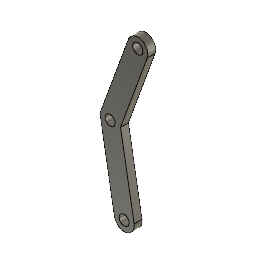
default (Autodesk Fusion 360 archive; units mm, degrees)
design "linkage2"
Autodesk Fusion 360 part; units mm, degrees
sketch "Sketch1" plane through (0, 0, 0) normal (0, 1, 0) x (1, 0, 0)
  line L0 (0, 0) -> (-735.0705, 0) construction
  line L1 (0, 0) -> (-636.5897, -367.5353) construction
  line L2 (0, 0) -> (-735.0705, -196.9616) construction
  circle A0 centre (-735.0705, -196.9616) radius 25
  circle A1 centre (-735.0705, -196.9616) radius 12.5
  circle A2 centre (-700.3409, 0) radius 25
  circle A3 centre (-700.3409, 0) radius 12.5
  circle A4 centre (-666.6665, -384.9001) radius 25
  circle A5 centre (-666.6665, -384.9001) radius 12.5
  line L3 (-675.7207, -4.3412) -> (-710.4503, -201.3028)
  line L4 (-759.6907, -192.6203) -> (-724.9611, 4.3412)
  line L5 (-643.1742, -376.3496) -> (-711.5782, -188.411)
  line L6 (-690.1588, -393.4506) -> (-758.5628, -205.5121)
  line L7 (-666.6665, -384.9001) -> (-735.0705, -196.9616) construction
  line L8 (-735.0705, -196.9616) -> (-700.3409, 0) construction
  line L9 (-735.0705, -196.9616) -> (-735.0705, 0) construction
  line L10 (-735.0705, -196.9616) -> (-636.5897, -367.5353) construction
  dimension "d2" = 30
  dimension "d3" = 15
  dimension "d6" = 50
  dimension "d7" = 25
  dimension "d8" = 50
  dimension "d9" = 25
  dimension "d10" = 50
  dimension "d11" = 25
  dimension "d15" = 10
  dimension "d16" = 10
  dimension "d17" = 200
  measures "d2" angle of L0 L1
  measures "d3" angle of L0 L2
  measures "d6" diameter of A0
  measures "d7" diameter of A1
  measures "d8" diameter of A4
  measures "d9" diameter of A5
  measures "d10" diameter of A2
  measures "d11" diameter of A3
  measures "d15" angle of L8 L9
  measures "d16" angle of L7 L10
extrude "Extrude1" add sketch "Sketch1" along normal mid plane 20
equation "d3 = d2 / 2"
equation "d7 = d6 / 2"
equation "d8 = d6"
equation "d9 = d7"
equation "d10 = d6"
equation "d11 = d7"
equation "d16 = d15"

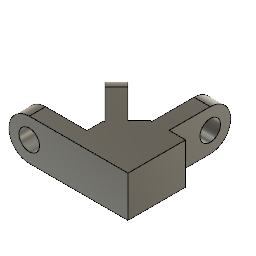
design "node2"
Autodesk Fusion 360 part; units mm, degrees
sketch "Sketch1" plane through (0, 0, 0) normal (0, 1, 0) x (1, 0, 0)
  circle A0 centre (-100, 0) radius 12.5
  circle A1 centre (100, 0) radius 12.5
  line L0 (100, 0) -> (-100, 0) construction
  circle A2 centre (-100, 0) radius 25
  circle A3 centre (100, 0) radius 25
  line L1 (100, -25) -> (-100, -25)
  line L2 (100, 25) -> (-100, 25)
  dimension "d1" = 200
  dimension "d2" = 25
  dimension "d3" = 25
  dimension "d4" = 12.5
  measures "d2" diameter of A0
  measures "d3" diameter of A1
  measures "d4" distance of A0 A2
extrude "Extrude1" add sketch "Sketch1" along normal mid plane 40 makes body 1
sketch "Sketch2" plane through (0, 0, 0) normal (1, 0, 0) x (0, 1, 0)
  circle A0 centre (100, 0) radius 12.5
  circle A1 centre (-100, 0) radius 12.5
  line L0 (100, 0) -> (-100, 0) construction
  circle A2 centre (-100, 0) radius 25
  circle A3 centre (100, 0) radius 25
  line L1 (100, 25) -> (-100, 25)
  line L2 (100, -25) -> (-100, -25)
  dimension "d8" = 200
  dimension "d9" = 25
  dimension "d10" = 25
  dimension "d11" = 12.5
  measures "d9" diameter of A1
  measures "d10" diameter of A0
  measures "d11" distance of A1 A2
extrude "Extrude2" add sketch "Sketch2" along normal mid plane 40 bodies 1
pattern_circular "C-Pattern1" count 2 over 45 about axis through (0, 0, 1.75) along (0, 0, 1) of bodies 1 makes body 2
sketch "Sketch3" plane through (0, 0, 0) normal (0, 0, 1) x (1, 0, 0)
  circle A0 centre (0, 0) radius 169.3734
  line L0 (20, -20) -> (-168.1884, -20)
  line L1 (20, -20) -> (20, 168.1884)
extrude "Extrude3" cut sketch "Sketch3" along normal mid plane 60 contours A0 L0 L1 picked at (28.044, 103.9038) bodies 1 2
combine "Combine1" operation add target body 1 tool bodies 2
sketch "Sketch4" plane through (0, 0, 0) normal (0, 1, 0) x (1, 0, 0)
  circle A0 centre (-100, 0) radius 25
  circle A1 centre (-100, 0) radius 12.5
  line L0 (-100, 25) -> (-50, 25)
  line L1 (-50, 25) -> (-50, -25)
  line L2 (-50, -25) -> (-100, -25)
  dimension "d18" = 50
  dimension "d19" = 50
  measures "d18" diameter of A0
extrude "Extrude4" cut sketch "Sketch4" along normal blind 20 bodies 1
pattern_circular "C-Pattern2" count 3 over 90 about axis through (0, 0, 1.75) along (0, 0, -1) of "Extrude4"
equation "d3 = d2"
equation "d8 = d1"
equation "d9 = d2"
equation "d10 = d2"
equation "d11 = d4"
equation "d18 = d2 + 2 * d4"
equation "d19 = 2 * d2"

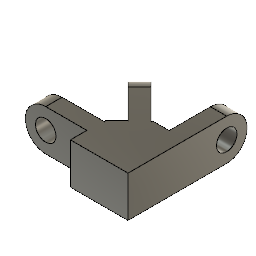
design "node1"
Autodesk Fusion 360 part; units mm, degrees
sketch "Sketch1" plane through (0, 0, 0) normal (0, 1, 0) x (1, 0, 0)
  circle A0 centre (-100, 0) radius 12.5
  circle A1 centre (100, 0) radius 12.5
  line L0 (100, 0) -> (-100, 0) construction
  circle A2 centre (-100, 0) radius 25
  circle A3 centre (100, 0) radius 25
  line L1 (100, -25) -> (-100, -25)
  line L2 (100, 25) -> (-100, 25)
  dimension "d1" = 200
  dimension "d2" = 25
  dimension "d3" = 25
  dimension "d4" = 12.5
  measures "d2" diameter of A0
  measures "d3" diameter of A1
  measures "d4" distance of A0 A2
extrude "Extrude1" add sketch "Sketch1" along normal mid plane 40 makes body 1
sketch "Sketch2" plane through (0, 0, 0) normal (1, 0, 0) x (0, 1, 0)
  circle A0 centre (100, 0) radius 12.5
  circle A1 centre (-100, 0) radius 12.5
  line L0 (100, 0) -> (-100, 0) construction
  circle A2 centre (-100, 0) radius 25
  circle A3 centre (100, 0) radius 25
  line L1 (100, 25) -> (-100, 25)
  line L2 (100, -25) -> (-100, -25)
  dimension "d8" = 200
  dimension "d9" = 25
  dimension "d10" = 25
  dimension "d11" = 12.5
  measures "d9" diameter of A1
  measures "d10" diameter of A0
  measures "d11" distance of A1 A2
extrude "Extrude2" add sketch "Sketch2" along normal mid plane 40 bodies 1
pattern_circular "C-Pattern1" count 2 over 45 about axis through (0, 0, 1.75) along (0, 0, 1) of bodies 1 makes body 2
sketch "Sketch3" plane through (0, 0, 0) normal (0, 0, 1) x (1, 0, 0)
  circle A0 centre (0, 0) radius 169.3734
  line L0 (20, -20) -> (-168.1884, -20)
  line L1 (20, -20) -> (20, 168.1884)
extrude "Extrude3" cut sketch "Sketch3" along normal mid plane 60 contours A0 L0 L1 picked at (28.044, 103.9038) bodies 1 2
combine "Combine1" operation add target body 1 tool bodies 2
sketch "Sketch4" plane through (0, 0, 0) normal (0, 1, 0) x (1, 0, 0)
  circle A0 centre (-100, 0) radius 25
  circle A1 centre (-100, 0) radius 12.5
  line L0 (-100, -25) -> (-50, -25)
  line L1 (-50, -25) -> (-50, 25)
  line L2 (-50, 25) -> (-100, 25)
  dimension "d18" = 50
  dimension "d19" = 50
  measures "d18" diameter of A0
extrude "Extrude4" cut sketch "Sketch4" against normal blind 20 bodies 1
pattern_circular "C-Pattern2" count 3 over 90 about axis through (0, 0, 1.75) along (0, 0, -1) of "Extrude4"
equation "d3 = d2"
equation "d8 = d1"
equation "d9 = d2"
equation "d10 = d2"
equation "d11 = d4"
equation "d18 = d2 + 2 * d4"
equation "d19 = 2 * d2"

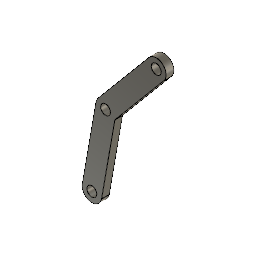
design "linkage1"
Autodesk Fusion 360 part; units mm, degrees
sketch "Sketch1" plane through (0, 0, 0) normal (0, 1, 0) x (1, 0, 0)
  line L0 (0, 0) -> (-735.0705, 0) construction
  line L1 (0, 0) -> (-636.5897, -367.5353) construction
  line L2 (0, 0) -> (-735.0705, -196.9616) construction
  circle A0 centre (-769.8001, 0) radius 25
  circle A1 centre (-606.513, -350.1704) radius 25
  circle A2 centre (-735.0705, -196.9616) radius 12.5
  circle A3 centre (-735.0705, -196.9616) radius 25
  line L3 (-759.6907, -201.3028) -> (-794.4203, -4.3412)
  line L4 (-710.4503, -192.6203) -> (-745.18, 4.3412)
  line L5 (-587.3619, -334.1007) -> (-715.9194, -180.8919)
  line L6 (-625.6641, -366.2401) -> (-754.2216, -213.0312)
  circle A4 centre (-769.8001, 0) radius 12.5
  circle A5 centre (-606.513, -350.1704) radius 12.5
  line L7 (-735.0705, 0) -> (-735.0705, -196.9616) construction
  line L8 (-636.5897, -367.5353) -> (-735.0705, -196.9616) construction
  line L9 (-735.0705, -196.9616) -> (-769.8001, 0) construction
  line L10 (-735.0705, -196.9616) -> (-606.513, -350.1704) construction
  dimension "d2" = 30
  dimension "d3" = 15
  dimension "d7" = 50
  dimension "d8" = 50
  dimension "d9" = 25
  dimension "d10" = 50
  dimension "d11" = 25
  dimension "d12" = 25
  dimension "d18" = 10
  dimension "d19" = 10
  dimension "d20" = 200
  measures "d2" angle of L0 L1
  measures "d3" angle of L0 L2
  measures "d7" diameter of A0
  measures "d8" diameter of A1
  measures "d9" diameter of A2
  measures "d10" diameter of A3
  measures "d11" diameter of A4
  measures "d12" diameter of A5
  measures "d18" angle of L7 L9
  measures "d19" angle of L8 L10
extrude "Extrude1" add sketch "Sketch1" along normal mid plane 20
equation "d2 = ( 90 / 3 ) * 1 deg"
equation "d3 = d2 / 2"
equation "d8 = d7"
equation "d9 = d7 / 2"
equation "d10 = d7"
equation "d11 = d9"
equation "d12 = d9"
equation "d19 = d18"
